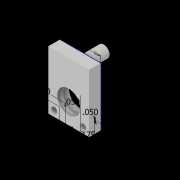
# Autodesk Inventor part: Slider
Saved by Autodesk Inventor 2017 (Build 210142000, 142)
## iProperties
Created: 2016-12-23
Part Number: Slider
Material: Generic
Document SubType Name: Modeling
Designer: David Kopala
Density: 1 g/cm^3
Appearance: Default
Author: David Kopala
Autodesk Inventor part; units mm, degrees
ref_plane "YZ Plane" through (0, 0, 0) normal (1, 0, 0) x (0, 1, 0)
ref_plane "XZ Plane" through (0, 0, 0) normal (0, 1, 0) x (-1, 0, 0)
ref_plane "XY Plane" through (0, 0, 0) normal (0, 0, 1) x (1, 0, 0)
sketch "Sketch1" plane through (0, 0, 0) normal (0, 0, 1) x (1, 0, 0)
  line L0 (0, 0) -> (8.89, 0)
  line L1 (8.89, 0) -> (8.89, 12.7)
  line L2 (8.89, 12.7) -> (0, 12.7)
  line L3 (0, 12.7) -> (0, 0)
  circle A0 centre (7.62, 1.27) radius 0.635
  circle A1 centre (1.27, 1.27) radius 0.635
  point P0 (4.445, 4.445)
  dimension "d0" = 8.89
  dimension "d1" = 12.7
  dimension "d18" = 1.27
  dimension "d19" = 1.27
  dimension "d20" = 1.27
  dimension "d21" = 1.27
  dimension "d22" = 1.27
  dimension "d23" = 1.27
  dimension "d26" = 4.445
  constraints: 8 end point, 2 centre point, 2 parallel, 1 horizontal, 1 perpendicular
  measures "d0" distance of L2.end L1.end
  measures "d1" distance of L1.end L0.end
  measures "d18" diameter of A0
  measures "d19" distance from line of L1 A0.centre
  measures "d20" distance from line of L0 A0.centre
  measures "d21" diameter of A1
  measures "d22" distance from line of A1.centre L3
  measures "d23" distance from line of A1.centre L0
  measures "d26" distance from line of L1 point (4.445, 4.445)
extrude "Extrusion1" add sketch "Sketch1" along normal blind 2.54 contours L3 L2 L1 L0 | A0 | A1
sketch "Sketch2" plane through (0, 0, 2.54) normal (0, 0, 1) x (1, 0, 0)
  circle A0 centre (4.445, 10.16) radius 1.27
  line L0 (8.89, 12.7) -> (0, 12.7) projected
  line L1 (8.89, 0) -> (8.89, 12.7) projected
  point P0 (0, 0)
  dimension "d5" = 2.54
  dimension "d6" = 2.54
  dimension "d7" = 4.445
  constraints: 1 centre point
  measures "d5" diameter of A0
  measures "d6" distance from line of L0 A0.centre
  measures "d7" distance from line of L1 A0.centre
extrude "Extrusion2" add sketch "Sketch2" against normal blind 7.62
hole "Hole1" at (4.445, 4.445, 0) direction (0, 0, 1) diameter 4.9784 depth 19.05 tip angle 118 thread size "1/4-20 UNC" class "2B" standard "ANSI Unified Screw Threads"
extrude "Extrusion3" cut sketch "Sketch1" along normal blind 5.08 contours A0 | A1
body "Solid1"
